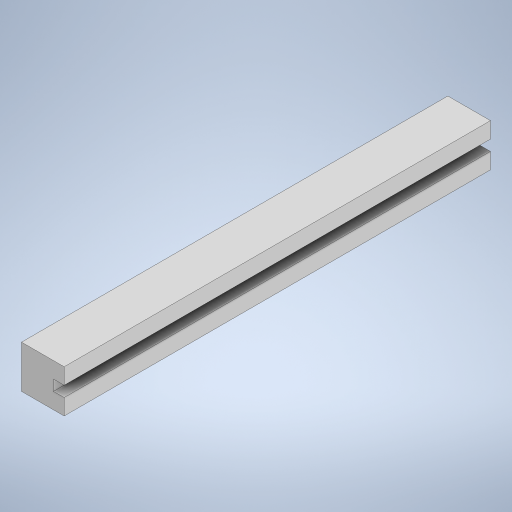
# Autodesk Inventor part: glass holder drawr X8
Saved by Autodesk Inventor 2023 (Build 270158000, 158)
## iProperties
Created: 2022-11-22
Part Number: glass holder drawr X8
Material: Generic
Document SubType Name: Modeling
Designer: surat
Density: 1 g/cm^3
Appearance: Default
Author: surat
Autodesk Inventor part; units mm, degrees
ref_plane "YZ Plane" through (0, 0, 0) normal (1, 0, 0) x (0, 1, 0)
ref_plane "XZ Plane" through (0, 0, 0) normal (0, 1, 0) x (-1, 0, 0)
ref_plane "XY Plane" through (0, 0, 0) normal (0, 0, 1) x (1, 0, 0)
sketch "Sketch1" plane through (0, 0, 0) normal (0, 1, 0) x (-1, 0, 0)
  line L0 (6.7607, 5.7456) -> (-18.6393, 5.7456)
  line L1 (-18.6393, 5.7456) -> (-18.6393, -248.2544)
  line L2 (-18.6393, -248.2544) -> (6.7607, -248.2544)
  line L3 (6.7607, -248.2544) -> (6.7607, 5.7456)
  point P0 (0, 0)
  dimension "d0" = 25.4
  dimension "d1" = 254
  constraints: 8 end point, 2 parallel, 1 horizontal, 1 perpendicular
  measures "d0" distance of L2.end L1.end
  measures "d1" distance of L1.end L0.end
extrude "Extrusion1" add sketch "Sketch1" along normal blind 25.4
sketch "Sketch2" plane through (18.6393, 0, 5.7456) normal (1, 0, 0) x (0, 0, -1)
  line L0 (0, 0) -> (0, 25.4) projected
  line L1 (254, 0) -> (254, 25.4) projected
  line L2 (0, 15.875) -> (254, 15.875)
  line L3 (254, 15.875) -> (254, 9.525)
  line L4 (254, 9.525) -> (0, 9.525)
  line L5 (0, 9.525) -> (0, 15.875)
  line L6 (0, 25.4) -> (254, 25.4) projected
  line L7 (0, 0) -> (254, 0) projected
  point P0 (5.7456, 0)
  point P1 (0, 9.525)
  dimension "d4" = 6.35
  dimension "d5" = 9.525
  constraints: 8 end point, 2 parallel, 2 point on line, 1 horizontal, 1 perpendicular
  measures "d4" distance between parallel lines of L4 L2
  measures "d5" distance between parallel lines of L2 L6
extrude "Extrusion2" cut sketch "Sketch2" against normal blind 6.35 contours L0 L2 L1 L4
sketch "Sketch3" plane through (-6.7607, 0, -248.2544) normal (-1, 0, 0) x (0, 0, 1)
  circle A0 centre (241.3, 12.7) radius 1.5875
  circle A1 centre (12.7, 12.7) radius 1.5875
  line L0 (0, 0) -> (0, 25.4) projected
  line L1 (0, 25.4) -> (254, 25.4) projected
  line L2 (254, 0) -> (254, 25.4) projected
  line L3 (0, 0) -> (254, 0) projected
  point P0 (248.2544, 0)
  dimension "d8" = 3.175
  dimension "d9" = 3.175
  dimension "d10" = 12.7
  dimension "d11" = 12.7
  dimension "d12" = 12.7
  dimension "d13" = 12.7
  constraints: 2 centre point
  measures "d8" diameter of A0
  measures "d9" diameter of A1
  measures "d10" distance from line of A1.centre L0
  measures "d11" distance from line of L1 A1.centre
  measures "d12" distance from line of L2 A0.centre
  measures "d13" distance from line of L3 A0.centre
extrude "Extrusion3" cut sketch "Sketch3" against normal blind 76.2 contours A0 | A1
chamfer "Chamfer1" distance 3.175 angle 45 2 edges at (-6.7607, 12.7, -237.1419) (-6.7607, 12.7, -8.5419)
body "Solid1"
